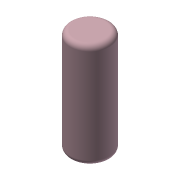
# Autodesk Inventor part: PP-14
Saved by Autodesk Inventor 2022 (Build 260148000, 148)
## iProperties
Created: 2008-09-23
Part Number: PP-14
Document SubType Name: Modeling
Designer: Mark Flayler
Mass: 0.121527 g
Surface Area: 1.51464 cm^2
Volume: 0.130674 cm^3
Density: 0.93 g/cm^3
Material: Rubber
Description: ERASER
Appearance: Pink Champagne
Author: Mark Flayler
Autodesk Inventor part; units mm, degrees
ref_plane "YZ Plane" through (0, 0, 0) normal (1, 0, 0) x (0, 1, 0)
ref_plane "XZ Plane" through (0, 0, 0) normal (0, 1, 0) x (-1, 0, 0)
ref_plane "XY Plane" through (0, 0, 0) normal (0, 0, 1) x (1, 0, 0)
sketch "Sketch1" plane through (0, 0, 0) normal (0, 0, 1) x (1, 0, 0)
  circle A0 centre (0, 0) radius 2
  dimension "d0" = 4
  constraints: 1 centre point, 1 coincident
  measures "d0" diameter of A0
extrude "Extrusion1" add sketch "Sketch1" along normal blind 10.5
fillet "Fillet1" radius 0.5 2 edges at (-2, 0, 0) (-2, 0, 10.5)
body "Solid1"
